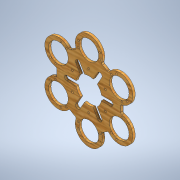
# Autodesk Inventor part: GenevaHolder
Saved by Autodesk Inventor 2020.2 (Build 242310000, 310)
## iProperties
Created: 2019-11-06
Part Number: GenevaHolder
Material: Plywood, Finish
Document SubType Name: Modeling
Designer: Paul Lefeuvre
Density: 0.552 g/cm^3
Appearance: Plywood - New
Author: Paul Lefeuvre
Autodesk Inventor part; units mm, degrees
ref_plane "YZ Plane" through (0, 0, 0) normal (1, 0, 0) x (0, 1, 0)
ref_plane "XZ Plane" through (0, 0, 0) normal (0, 1, 0) x (-1, 0, 0)
ref_plane "XY Plane" through (0, 0, 0) normal (0, 0, 1) x (1, 0, 0)
sketch "Sketch1" plane through (0, 0, 0) normal (0, 0, 1) x (1, 0, 0)
  circle A0 centre (0, 0) radius 175 construction
  line L0 (0, 0) -> (0, 152.9684) construction
  circle A1 centre (0, 0) radius 50
  line L1 (0, 0) -> (-42.671, 73.9083)
  line L2 (-31.9973, 38.421) -> (-50.0322, 69.6583)
  line L3 (-17.2749, 46.921) -> (-35.3098, 78.1583)
  arc A2 (-35.3098, 78.1583) -> (-50.0322, 69.6583) centre (-42.671, 73.9083) ccw
  line L4 (-16.7016, 47.1281) -> (-34.7901, 78.4583)
  arc A3 (-34.7901, 78.4583) -> (-50.5518, 69.3583) centre (-42.671, 73.9083) ccw
  line L5 (-50.5518, 69.3583) -> (-32.4633, 38.0281)
  line L6 (-49.1649, 9.1) -> (-85.342, 9.1)
  arc A4 (-85.342, 9.1) -> (-85.342, -9.1) centre (-85.342, 0) ccw
  line L7 (-85.342, -9.1) -> (-49.1649, -9.1)
  line L8 (-49.2722, 8.5) -> (-85.342, 8.5)
  arc A5 (-85.342, 8.5) -> (-85.342, -8.5) centre (-85.342, 0) ccw
  line L9 (-49.2722, -8.5) -> (-85.342, -8.5)
  line L10 (-32.4633, -38.0281) -> (-50.5518, -69.3583)
  arc A6 (-50.5518, -69.3583) -> (-34.7901, -78.4583) centre (-42.671, -73.9083) ccw
  line L11 (-34.7901, -78.4583) -> (-16.7016, -47.1281)
  line L12 (-31.9973, -38.421) -> (-50.0322, -69.6583)
  arc A7 (-50.0322, -69.6583) -> (-35.3098, -78.1583) centre (-42.671, -73.9083) ccw
  line L13 (-17.2749, -46.921) -> (-35.3098, -78.1583)
  line L14 (16.7016, -47.1281) -> (34.7901, -78.4583)
  arc A8 (34.7901, -78.4583) -> (50.5518, -69.3583) centre (42.671, -73.9083) ccw
  line L15 (50.5518, -69.3583) -> (32.4633, -38.0281)
  line L16 (17.2749, -46.921) -> (35.3098, -78.1583)
  arc A9 (35.3098, -78.1583) -> (50.0322, -69.6583) centre (42.671, -73.9083) ccw
  line L17 (31.9973, -38.421) -> (50.0322, -69.6583)
  line L18 (49.1649, -9.1) -> (85.342, -9.1)
  arc A10 (85.342, -9.1) -> (85.342, 9.1) centre (85.342, 0) ccw
  line L19 (85.342, 9.1) -> (49.1649, 9.1)
  line L20 (49.2722, -8.5) -> (85.342, -8.5)
  arc A11 (85.342, -8.5) -> (85.342, 8.5) centre (85.342, 0) ccw
  line L21 (49.2722, 8.5) -> (85.342, 8.5)
  line L22 (32.4633, 38.0281) -> (50.5518, 69.3583)
  arc A12 (50.5518, 69.3583) -> (34.7901, 78.4583) centre (42.671, 73.9083) ccw
  line L23 (34.7901, 78.4583) -> (16.7016, 47.1281)
  line L24 (31.9973, 38.421) -> (50.0322, 69.6583)
  arc A13 (50.0322, 69.6583) -> (35.3098, 78.1583) centre (42.671, 73.9083) ccw
  line L25 (17.2749, 46.921) -> (35.3098, 78.1583)
  arc A14 (49.2722, -8.5) -> (17.2749, 46.921) centre (49.2722, 28.4473) ccw construction
  circle A15 centre (0, 0) radius 93.842 construction
  arc A16 (17.2749, 46.921) -> (49.2722, -8.5) centre (49.2722, 28.4473) ccw construction
  circle A17 centre (49.2722, 28.4473) radius 19.9473 construction
  circle A18 centre (0, 0) radius 74.4 construction
  circle A19 centre (0, 74.4) radius 3.9
  circle A20 centre (-64.4323, 37.2) radius 3.9
  circle A21 centre (-64.4323, -37.2) radius 3.9
  circle A22 centre (0, -74.4) radius 3.9
  circle A23 centre (64.4323, -37.2) radius 3.9
  circle A24 centre (64.4323, 37.2) radius 3.9
  circle A25 centre (0, 136.9) radius 38.1
  circle A26 centre (0, 136.9) radius 37.5 construction
  arc A27 (-52.7754, 113.3126) -> (-71.7439, 102.3612) centre (0, 0) ccw
  arc A28 (-124.5193, 10.9515) -> (-124.5193, -10.9515) centre (0, 0) ccw
  arc A29 (-71.7439, -102.3612) -> (-52.7754, -113.3126) centre (0, 0) ccw
  arc A30 (52.7754, -113.3126) -> (71.7439, -102.3612) centre (0, 0) ccw
  arc A31 (124.5193, -10.9515) -> (124.5193, 10.9515) centre (0, 0) ccw
  arc A32 (71.7439, 102.3612) -> (52.7754, 113.3126) centre (0, 0) ccw
  arc A33 (50.163, 119.485) -> (-50.163, 119.485) centre (0, 136.9) ccw
  arc A34 (-52.7754, 113.3126) -> (-50.163, 119.485) centre (-54.8865, 117.8451) ccw
  arc A35 (50.163, 119.485) -> (52.7754, 113.3126) centre (54.8865, 117.8451) ccw
  arc A36 (-78.3955, 103.1849) -> (-128.5585, 16.3001) centre (-118.5589, 68.45) ccw
  circle A37 centre (-118.5589, 68.45) radius 38.1
  arc A38 (-78.3955, 103.1849) -> (-71.7439, 102.3612) centre (-74.6137, 106.4556) ccw
  arc A39 (-124.5193, 10.9515) -> (-128.5585, 16.3001) centre (-129.5001, 11.3895) ccw
  arc A40 (-128.5585, -16.3001) -> (-78.3955, -103.1849) centre (-118.5589, -68.45) ccw
  circle A41 centre (-118.5589, -68.45) radius 38.1
  arc A42 (-128.5585, -16.3001) -> (-124.5193, -10.9515) centre (-129.5001, -11.3895) ccw
  arc A43 (-71.7439, -102.3612) -> (-78.3955, -103.1849) centre (-74.6137, -106.4556) ccw
  arc A44 (-50.163, -119.485) -> (50.163, -119.485) centre (0, -136.9) ccw
  circle A45 centre (0, -136.9) radius 38.1
  arc A46 (-50.163, -119.485) -> (-52.7754, -113.3126) centre (-54.8865, -117.8451) ccw
  arc A47 (52.7754, -113.3126) -> (50.163, -119.485) centre (54.8865, -117.8451) ccw
  arc A48 (78.3955, -103.1849) -> (128.5585, -16.3001) centre (118.5589, -68.45) ccw
  circle A49 centre (118.5589, -68.45) radius 38.1
  arc A50 (78.3955, -103.1849) -> (71.7439, -102.3612) centre (74.6137, -106.4556) ccw
  arc A51 (124.5193, -10.9515) -> (128.5585, -16.3001) centre (129.5001, -11.3895) ccw
  arc A52 (128.5585, 16.3001) -> (78.3955, 103.1849) centre (118.5589, 68.45) ccw
  circle A53 centre (118.5589, 68.45) radius 38.1
  arc A54 (128.5585, 16.3001) -> (124.5193, 10.9515) centre (129.5001, 11.3895) ccw
  arc A55 (71.7439, 102.3612) -> (78.3955, 103.1849) centre (74.6137, 106.4556) ccw
  circle A56 centre (41.5415, 148.9) radius 3.3
  circle A57 centre (41.5415, 124.9) radius 3.3
  line L26 (0, 136.9) -> (41.5415, 148.9) construction
  line L27 (41.5415, 148.9) -> (41.5415, 124.9) construction
  line L28 (41.5415, 124.9) -> (0, 136.9) construction
  circle A58 centre (-41.5415, 148.9) radius 3.3
  circle A59 centre (-41.5415, 124.9) radius 3.3
  circle A60 centre (-108.1804, 110.426) radius 3.3
  circle A61 centre (-87.3958, 98.426) radius 3.3
  circle A62 centre (-149.7219, 38.474) radius 3.3
  circle A63 centre (-128.9373, 26.474) radius 3.3
  circle A64 centre (-149.7219, -38.474) radius 3.3
  circle A65 centre (-128.9373, -26.474) radius 3.3
  circle A66 centre (-108.1804, -110.426) radius 3.3
  circle A67 centre (-87.3958, -98.426) radius 3.3
  circle A68 centre (-41.5415, -148.9) radius 3.3
  circle A69 centre (-41.5415, -124.9) radius 3.3
  circle A70 centre (41.5415, -148.9) radius 3.3
  circle A71 centre (41.5415, -124.9) radius 3.3
  circle A72 centre (108.1804, -110.426) radius 3.3
  circle A73 centre (87.3958, -98.426) radius 3.3
  circle A74 centre (149.7219, -38.474) radius 3.3
  circle A75 centre (128.9373, -26.474) radius 3.3
  circle A76 centre (149.7219, 38.474) radius 3.3
  circle A77 centre (128.9373, 26.474) radius 3.3
  circle A78 centre (108.1804, 110.426) radius 3.3
  circle A79 centre (87.3958, 98.426) radius 3.3
  point P0 (49.2722, -8.5)
  point P1 (31.9973, -38.421)
  point P2 (17.2749, -46.921)
  point P3 (-17.2749, -46.921)
  point P4 (-31.9973, -38.421)
  point P5 (-49.2722, -8.5)
  point P6 (17.2749, 46.921)
  point P7 (31.9973, 38.421)
  point P8 (49.2722, 8.5)
  point P9 (-34.3824, 120.4848)
  point P10 (-32.4194, 116.8852)
  point P11 (34.2525, 120.2155)
  point P12 (32.4194, 116.8852)
  point P13 (-85.0158, 86.5186)
  point P14 (-117.4353, 30.3666)
  point P15 (-121.5341, 30.4663)
  point P16 (-86.9834, 89.7713)
  point P17 (-117.4353, -30.3666)
  point P18 (-85.0158, -86.5186)
  point P19 (-87.1517, -90.0184)
  point P20 (-121.2359, -30.4442)
  point P21 (-32.4194, -116.8852)
  point P22 (32.4194, -116.8852)
  point P23 (34.3824, -120.4848)
  point P24 (-34.2525, -120.2155)
  point P25 (85.0158, -86.5186)
  point P26 (117.4353, -30.3666)
  point P27 (121.5341, -30.4663)
  point P28 (86.9834, -89.7713)
  point P29 (117.4353, 30.3666)
  point P30 (85.0158, 86.5186)
  point P31 (87.1517, 90.0184)
  point P32 (121.2359, 30.4442)
  dimension "d2" = 100
  dimension "d26" = 148.8
  dimension "d0" = 350
  dimension "d3" = 30
  dimension "d4" = 17
  dimension "d5" = 0.6
  dimension "d8" = 360
  dimension "d27" = 7.8
  dimension "d30" = 360
  dimension "d42" = 0.6
  dimension "d43" = 125
  dimension "d44" = 75
  dimension "d45" = 15
  dimension "d48" = 5
  dimension "d51" = 360
  dimension "d53" = 6.6
  dimension "d54" = 6.6
  dimension "d56" = 43.24
  dimension "d57" = 24
  dimension "d58" = 43.24
  dimension "d61" = 360
  constraints: 100 point on circle, 77 centre point, 58 end point, 12 tangent, 11 coincident, 6 equal radius, 3 parallel, 2 point on line, 2 symmetric about line, 2 vertical, 1 vertical alignment, 260 other
  measures "d0" diameter of A0
  measures "d3" angle of L0 L1
  measures "d4" distance between parallel lines of L2 L3
  measures "d5" distance between parallel lines of L3 L4
  measures "d27" diameter of A19
  measures "d42" radial gap between concentric circles of A25 A26
  measures "d43" radius of A32
  measures "d44" diameter of A26
  measures "d45" radial gap between concentric circles of A25 A33
  measures "d48" radius of A34
  measures "d53" diameter of A56
  measures "d54" diameter of A57
  measures "d56" distance of L26.start L26.end
  measures "d57" distance of L26.end L27.end
  measures "d58" distance of L27.end L28.end
extrude "Extrusion1" add sketch "Sketch1" along normal blind 9
body "Solid1"
